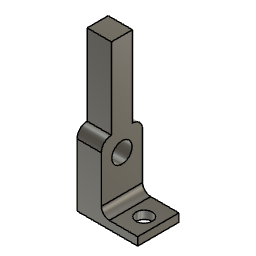
End-Axle Supports (Autodesk Fusion 360 design; units mm, degrees)
Autodesk Fusion 360 part; units mm, degrees
sketch "Sketch1" plane through (0, 0, 0) normal (0, 0, 1) x (1, 0, 0)
  line L0 (0, 0) -> (32, 0)
  line L1 (32, 0) -> (32, 10.2)
  line L2 (32, 10.2) -> (0, 10.2)
  line L3 (0, 10.2) -> (0, 0)
  dimension "d1" = 32
  dimension "d2" = 10.2
  constraint horizontal L0
  constraint vertical L1
  constraint horizontal L2
  constraint vertical L3
  constraint coincident L0.start L3.end
  measures "d1" distance of L1 L3
  measures "d2" distance of L0 L2
extrude "Extrude1" add sketch "Sketch1" along normal blind 2
sketch "Sketch2" plane through (0, 0, 2) normal (0, 0, 1) x (-1, 0, 0)
  line L0 (0, -10.2) -> (0, 0)
  line L1 (0, 0) -> (-32, 0)
  line L2 (-32, 0) -> (-32, -10.2)
  line L3 (-32, -10.2) -> (0, -10.2)
  line L4 (-7, -10.2) -> (-25, -10.2)
  line L5 (-25, -10.2) -> (-25, 0)
  line L6 (-25, 0) -> (-7, 0)
  line L7 (-7, 0) -> (-7, -10.2)
  circle A0 centre (-3.5, -5.1) radius 2
  circle A1 centre (-28.5, -5.1) radius 2
  dimension "d5" = 7
  dimension "d6" = 7
  dimension "d7" = 5.1
  dimension "d8" = 3.5
  dimension "d9" = 4
  dimension "d10" = 3.5
  dimension "d11" = 5.1
  dimension "d12" = 4
  constraint horizontal L4
  constraint vertical L5
  constraint horizontal L6
  constraint vertical L7
  constraint coincident L1 L5.end
  constraint coincident L3 L4.start
  measures "d5" distance of L0 L7
  measures "d6" distance of L2 L5
  measures "d7" distance of L3 A0.centre
  measures "d8" distance of L7 A0.centre
  measures "d9" diameter of A0
  measures "d10" distance of L2 A1.centre
  measures "d11" distance of L1 A1.centre
  measures "d12" diameter of A1
extrude "Extrude2" cut sketch "Sketch2" against normal blind 2.1 contours A0 | A1
extrude "Extrude3" add sketch "Sketch2" along normal blind 16 contours L1 L3 L4 L5 L6 L7
sketch "Sketch3" plane through (25, 0, 0) normal (1, 0, 0) x (0, 1, 0)
  line L0 (0, 2) -> (10.2, 2)
  line L1 (10.2, 2) -> (10.2, 18)
  line L2 (10.2, 18) -> (0, 18)
  line L3 (0, 18) -> (0, 2)
  circle A0 centre (5.1, 13) radius 2.5
  dimension "d17" = 5
  dimension "d18" = 5.1
  dimension "d19" = 5
  measures "d17" distance of L2 A0.centre
  measures "d18" distance of L3 A0.centre
  measures "d19" diameter of A0
extrude "Extrude4" cut sketch "Sketch3" against normal blind 20 contours A0
fillet "Fillet1" radius 2.5 2 edges at (16, 0, 18) (16, 10.2, 18)
fillet "Fillet2" radius 0.25 2 edges at (25, 5.1, 2) (7, 5.1, 2)
sketch "Sketch4" plane through (0, 0, 0) normal (0, -1, 0) x (1, 0, 0)
  line L0 (25, 15.5) -> (7, 15.5)
  line L1 (7, 15.5) -> (7, 2.25)
  arc A0 (6.75, 2) -> (7, 2.25) centre (6.75, 2.25) ccw
  line L2 (6.75, 2) -> (0, 2)
  line L3 (0, 2) -> (0, 0)
  line L4 (0, 0) -> (32, 0)
  line L5 (32, 0) -> (32, 2)
  line L6 (32, 2) -> (25.25, 2)
  arc A1 (25, 2.25) -> (25.25, 2) centre (25.25, 2.25) ccw
  line L7 (25, 2.25) -> (25, 15.5)
  line L8 (15.0115, 13.8918) -> (15.2499, 13.8388)
  line L9 (15.0115, 1.9217) -> (15.2499, 1.8688)
  line L10 (15.2499, 2.3085) -> (10.5625, 8.1981)
  line L11 (10.6841, 8.3354) -> (15.2499, 13.4918)
  line L12 (10.817, 8.3354) -> (15.3124, 13.4128)
  line L13 (15.3132, 2.3954) -> (10.6954, 8.1981)
  spline S0 degree 5 poles (15.0115, 13.8918) (15.0366, 13.8331) (15.0755, 13.7537) (15.1214, 13.6739) (15.1743, 13.5935) (15.2341, 13.5126) (15.2499, 13.4918) knots 0 0 0 0 0 0 0.04 0.053771 0.053771 0.053771 0.053771 0.053771 0.053771
  line L14 (15.2177, 13.5342) -> (15.2821, 13.4495)
  spline S1 degree 5 poles (15.2499, 2.3085) (15.2476, 2.3054) (15.194, 2.2294) (15.1434, 2.1527) (15.0959, 2.0753) (15.0514, 1.9972) (15.0115, 1.9217) knots 0.958261 0.958261 0.958261 0.958261 0.958261 0.958261 0.96 1 1 1 1 1 1
  line L15 (15.2777, 2.3478) -> (15.2221, 2.2693)
  line L16 (19.8903, 8.1981) -> (19.6849, 7.759)
  line L17 (19.6849, 7.759) -> (20.8035, 8.2887)
  line L18 (20.8035, 8.2887) -> (19.6849, 8.7197)
  line L19 (19.6849, 8.7197) -> (19.8674, 8.3354)
  spline S2 degree 5 poles (15.2499, 13.8388) (15.275, 13.7801) (15.3328, 13.6621) (15.4428, 13.4833) (15.636, 13.2415) (15.9534, 12.9319) (16.3409, 12.6103) (16.7857, 12.2676) (17.2659, 11.8886) (17.7534, 11.4561) (18.2174, 10.9546) (18.6276, 10.3741) (18.9469, 9.734) (19.126, 9.1768) (19.2132, 8.7476) (19.2502, 8.4653) (19.263, 8.3354) knots 0 0 0 0 0 0 0.04 0.08 0.12 0.16 0.2 0.24 0.28 0.32 0.36 0.4 0.44 0.473865 0.473865 0.473865 0.473865 0.473865 0.473865
  line L20 (19.1848, 9.1287) -> (19.3411, 7.542)
  spline S3 degree 5 poles (19.2746, 8.1981) (19.2853, 8.0482) (19.2958, 7.7438) (19.2774, 7.2862) (19.1846, 6.69) (18.9625, 5.9984) (18.6463, 5.3801) (18.2572, 4.8452) (17.8198, 4.3863) (17.3603, 3.9873) (16.904, 3.6275) (16.4734, 3.2862) (16.0845, 2.9471) (15.7463, 2.6009) (15.5197, 2.3146) (15.375, 2.094) (15.2897, 1.9443) (15.2499, 1.8688) knots 0.481014 0.481014 0.481014 0.481014 0.481014 0.481014 0.52 0.56 0.6 0.64 0.68 0.72 0.76 0.8 0.84 0.88 0.92 0.96 1 1 1 1 1 1
  line L21 (19.2097, 9.1087) -> (19.3396, 7.2875)
  spline S4 degree 5 poles (15.3124, 13.4128) (15.332, 13.3889) (15.4036, 13.3041) (15.5393, 13.1573) (15.762, 12.9459) (16.1025, 12.6633) (16.5474, 12.3206) (17.0276, 11.9416) (17.515, 11.5091) (17.979, 11.0075) (18.3892, 10.427) (18.7131, 9.7778) (18.894, 9.2098) (18.9811, 8.7693) (19.0172, 8.476) (19.0296, 8.3354) knots 0.064218 0.064218 0.064218 0.064218 0.064218 0.064218 0.08 0.12 0.16 0.2 0.24 0.28 0.32 0.36 0.4 0.44 0.476625 0.476625 0.476625 0.476625 0.476625 0.476625
  line L22 (14.9219, 13.8881) -> (15.7028, 12.9376)
  line L23 (18.9651, 9.0672) -> (19.094, 7.6035)
  spline S5 degree 5 poles (19.0398, 8.1981) (19.0483, 8.0587) (19.0561, 7.765) (19.0358, 7.3185) (18.9432, 6.7334) (18.7242, 6.0513) (18.408, 5.433) (18.0189, 4.8982) (17.5814, 4.4393) (17.1219, 4.0403) (16.6657, 3.6805) (16.235, 3.3392) (15.8681, 3.0192) (15.6141, 2.7622) (15.4485, 2.5703) (15.3521, 2.4471) (15.3132, 2.3954) knots 0.483768 0.483768 0.483768 0.483768 0.483768 0.483768 0.52 0.56 0.6 0.64 0.68 0.72 0.76 0.8 0.84 0.88 0.92 0.948678 0.948678 0.948678 0.948678 0.948678 0.948678
  line L24 (18.989, 9.0312) -> (19.0905, 7.3649)
  line L25 (15.7537, 2.9821) -> (14.8727, 1.8087)
  line L26 (10.6954, 8.1981) -> (19.0398, 8.1981)
  line L27 (19.2746, 8.1981) -> (19.8903, 8.1981)
  line L28 (19.263, 8.3354) -> (19.8674, 8.3354)
  line L29 (10.6725, 8.3354) -> (10.3002, 8.665)
  line L30 (10.3002, 8.665) -> (9.1473, 8.665)
  line L31 (9.1473, 8.665) -> (9.409, 8.2777)
  line L32 (9.409, 8.2777) -> (9.1615, 7.917)
  line L33 (9.1615, 7.917) -> (10.3, 7.917)
  line L34 (10.3, 7.917) -> (10.5625, 8.1981)
  line L35 (10.6725, 8.3354) -> (10.6841, 8.3354)
  line L36 (10.817, 8.3354) -> (19.0296, 8.3354)
  point P0 (16.3357, 12.6206)
  point P1 (16.627, 3.4048)
  point P2 (18.7456, 10.1048)
  point P3 (18.825, 5.7617)
  point P4 (18.5867, 5.8147)
  point P5 (18.5072, 10.1578)
  point P6 (16.0973, 12.6736)
  point P7 (16.3886, 3.4577)
  constraint parallel L8 L9
  constraint midpoint L11.end L14
  constraint midpoint L10.start L15
  constraint horizontal L26
  constraint horizontal L35
  constraint coincident S2.end L35
  constraint midpoint S2.end L20
  constraint coincident S3.start L26
  constraint midpoint S3.start L21
  constraint midpoint L12.end L22
  constraint midpoint S4.end L23
  constraint midpoint S5.start L24
  constraint midpoint L13.start L25
  constraint collinear L26 L27
  constraint collinear L28 L35
  constraint perpendicular L11 L29
  constraint parallel L30 L35
  constraint horizontal L33
  constraint coincident L12.start L35
  constraint collinear L35 L36
extrude "Extrude5" cut sketch "Sketch4" against normal blind 0.3 contours L8 L9 S0 L14 S1 L15 S2 L20 S3 L21 S4 L22 L23 S5 L24 L25 | L16 L17 L18 L19 L20 L21 L27 L28 | L10 L11 L12 L13 L14 L15 L22 L23 L24 L25 L26 L29 L30 L31 L32 L33 L34 L35 L36
sketch "Sketch5" plane through (0, 0, 0) normal (0, -1, 0) x (1, 0, 0)
  line L0 (7, 15.5) -> (23, 15.5)
  line L1 (23, 15.5) -> (23, 0)
  line L2 (23, 0) -> (7, 0)
  line L3 (7, 0) -> (7, 15.5)
  line L4 (32, 0) -> (0, 0)
  point P0 (7, 15.5)
  constraint horizontal L0
  constraint vertical L1
  constraint horizontal L2
  constraint vertical L3
  constraint coincident L1.end L4
  constraint coincident P0 L0.start
extrude "Extrude6" add sketch "Sketch4" sketch "Sketch5" against normal blind 1 contours L0 L1 A0 L2 L3 L4 L5 L6 A1 L7 | L8 L9 S0 L14 S1 L15 S2 L20 S3 L21 S4 L22 L23 S5 L24 L25 | L16 L17 L18 L19 L20 L21 L27 L28 | L10 L11 L12 L13 L14 L15 L22 L23 L24 L25 L26 L29 L30 L31 L32 L33 L34 L35 L36 | L13 S5 L26 of sketch 2
sketch "Sketch6" plane through (0, 0, 0) normal (0, -1, 0) x (1, 0, 0)
  line L0 (25, 15.5) -> (7, 15.5)
  line L1 (7, 15.5) -> (7, 2.25)
  arc A0 (6.75, 2) -> (7, 2.25) centre (6.75, 2.25) ccw
  line L2 (6.75, 2) -> (0, 2)
  line L3 (0, 2) -> (0, 0)
  line L4 (0, 0) -> (32, 0)
  line L5 (32, 0) -> (32, 2)
  line L6 (32, 2) -> (25.25, 2)
  arc A1 (25, 2.25) -> (25.25, 2) centre (25.25, 2.25) ccw
  line L7 (25, 2.25) -> (25, 15.5)
  line L8 (0, 20) -> (17, 20)
  line L9 (17, 20) -> (17, 0)
  line L10 (17, 0) -> (0, 0)
  line L11 (0, 0) -> (0, 20)
  dimension "d32" = 17
  constraint horizontal L8
  constraint vertical L9
  constraint horizontal L10
  constraint vertical L11
  constraint coincident L4 L9.end
  measures "d32" distance of L9 L11
extrude "Extrude7" cut sketch "Sketch6" against normal blind 12 contours L0 L1 A0 L2 L3 L4 L9 L10 L11 | L0 L1 A0 L2 L8 L9 L11
sketch "Sketch7" plane through (0, 0, 0) normal (0, -1, 0) x (1, 0, 0)
  line L0 (17, 15.5) -> (17, 0)
  line L1 (17, 0) -> (32, 0)
  line L2 (32, 0) -> (32, 2)
  line L3 (32, 2) -> (25.25, 2)
  arc A0 (25, 2.25) -> (25.25, 2) centre (25.25, 2.25) ccw
  line L4 (25, 2.25) -> (25, 15.5)
  line L5 (25, 15.5) -> (17, 15.5)
  line L6 (23, 18) -> (25.1716, 18)
  line L7 (25.1716, 18) -> (25.1716, 2)
  line L8 (25.1716, 2) -> (23, 2)
  line L9 (23, 2) -> (23, 18)
  line L10 (25, 18) -> (17, 18)
  dimension "d35" = 2
  constraint horizontal L6
  constraint vertical L7
  constraint horizontal L8
  constraint vertical L9
  constraint coincident L3 L7.end
  constraint coincident L6.start L10
  measures "d35" distance of L4 L9
extrude "Extrude8" cut sketch "Sketch7" against normal blind 12 contours A0 L4 L5 L6 L7 L9 L10 | A0 L4 L5 L7 L8 L9
sketch "Sketch8" plane through (0, 10.2, 0) normal (0, 1, 0) x (-1, 0, 0)
  line L0 (-23, 15.5) -> (-23, 2)
  line L1 (-23, 2) -> (-25.1716, 2)
  line L2 (-25.1716, 2) -> (-25.1716, 2.0126)
  arc A0 (-25.25, 2) -> (-25.1716, 2.0126) centre (-25.25, 2.25) ccw
  line L3 (-25.25, 2) -> (-32, 2)
  line L4 (-32, 2) -> (-32, 0)
  line L5 (-32, 0) -> (-17, 0)
  line L6 (-17, 0) -> (-17, 15.5)
  line L7 (-17, 15.5) -> (-23, 15.5)
  line L8 (-25.2855, 2) -> (-25.1, 2)
  line L9 (-25.1, 2) -> (-25.1, 2.05)
  line L10 (-25.1, 2.05) -> (-25.2855, 2.05)
  line L11 (-25.2855, 2.05) -> (-25.2855, 2)
  constraint horizontal L8
  constraint vertical L9
  constraint horizontal L10
  constraint vertical L11
  constraint coincident L3 L8.start
extrude "Extrude9" cut sketch "Sketch8" against normal blind 12 contours L1 L2 A0 L3 L8 L9 L10 L11 | L2 A0 L8
fillet "Fillet3" radius 2 1 edges at (23, 5.1, 2)
extrude "Extrude10" add 1 faces at (21, 4.2333, 18) along direction (0, 0, 1) blind 20
